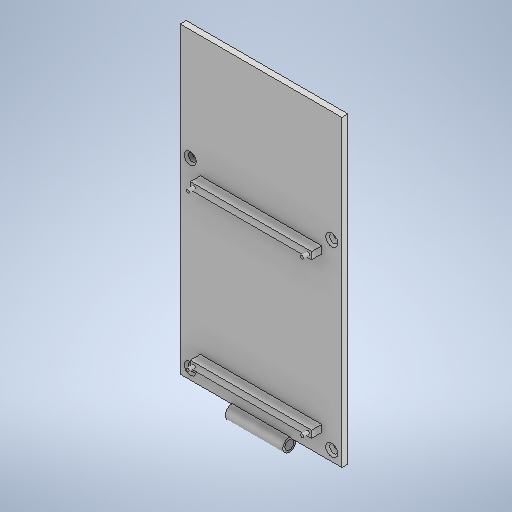
# Autodesk Inventor part: Backboard deel 1
Saved by Autodesk Inventor 2025.2 (Build 292293000, 293)
## iProperties
Created: 2024-12-12
Part Number: Backboard deel 1
Material: Generic
Document SubType Name: Modeling
Designer: jurre
Density: 1 g/cm^3
Appearance: Default
Author: jurre
Autodesk Inventor part; units mm, degrees
ref_plane "YZ Plane" through (0, 0, 0) normal (1, 0, 0) x (0, 1, 0)
ref_plane "XZ Plane" through (0, 0, 0) normal (0, 1, 0) x (-1, 0, 0)
ref_plane "XY Plane" through (0, 0, 0) normal (0, 0, 1) x (1, 0, 0)
sketch "Sketch1" plane through (0, 0, 0) normal (0, 0, 1) x (1, 0, 0)
  line L0 (-54.9903, 21.6893) -> (25.0097, 21.6893)
  line L1 (25.0097, 21.6893) -> (25.0097, -78.3107)
  line L2 (25.0097, -78.3107) -> (-54.9903, -78.3107)
  line L3 (-54.9903, -78.3107) -> (-54.9903, 21.6893)
  line L4 (-44.9903, 11.6893) -> (15.0097, 11.6893)
  line L5 (15.0097, 11.6893) -> (15.0097, -68.3107)
  line L6 (15.0097, -68.3107) -> (-44.9903, -68.3107)
  line L7 (-44.9903, -68.3107) -> (-44.9903, 11.6893)
  circle A0 centre (13.2597, 9.9393) radius 0.75
  circle A1 centre (-43.2403, 9.9393) radius 0.75
  circle A2 centre (-43.2403, -66.5607) radius 0.75
  circle A3 centre (13.2597, -66.5607) radius 0.75
  line L8 (-44.9903, 11.6893) -> (15.0097, 11.6893)
  line L9 (15.0097, 11.6893) -> (15.0097, 8.1893)
  line L10 (15.0097, 8.1893) -> (-44.9903, 8.1893)
  line L11 (-44.9903, 8.1893) -> (-44.9903, 11.6893)
  line L12 (15.0097, -68.3107) -> (-44.9903, -68.3107)
  line L13 (-44.9903, -68.3107) -> (-44.9903, -64.8107)
  line L14 (-44.9903, -64.8107) -> (15.0097, -64.8107)
  line L15 (15.0097, -64.8107) -> (15.0097, -68.3107)
  circle A4 centre (-49.9903, 16.6893) radius 2
  circle A5 centre (20.0097, 16.6893) radius 2
  circle A6 centre (20.0097, -73.3107) radius 2
  circle A7 centre (-49.9903, -73.3107) radius 2
  line L16 (-54.9903, 71.6893) -> (25.0097, 71.6893)
  line L17 (25.0097, 71.6893) -> (25.0097, -78.3107)
  line L18 (25.0097, -78.3107) -> (-54.9903, -78.3107)
  line L19 (-54.9903, -78.3107) -> (-54.9903, 71.6893)
  point P0 (0, 0)
  point P1 (-14.9903, -78.3107)
  point P2 (15.0097, -64.8107)
  point P3 (25.0097, 21.6893)
  dimension "d0" = 80
  dimension "d1" = 100
  dimension "d2" = 60
  dimension "d3" = 80
  dimension "d4" = 10
  dimension "d5" = 10
  dimension "d6" = 1.5
  dimension "d7" = 1.5
  dimension "d8" = 1.5
  dimension "d9" = 1.5
  dimension "d11" = 1.75
  dimension "d12" = 1.75
  dimension "d13" = 1.75
  dimension "d14" = 1.75
  dimension "d15" = 1.75
  dimension "d16" = 1.75
  dimension "d17" = 1.75
  dimension "d18" = 1.75
  dimension "d19" = 60
  dimension "d20" = 0
  dimension "d21" = 0
  dimension "d22" = 3.5
  dimension "d23" = 60
  dimension "d24" = 0
  dimension "d25" = 3.5
  dimension "d26" = 0
  dimension "d39" = 4
  dimension "d40" = 5
  dimension "d41" = 5
  dimension "d42" = 4
  dimension "d43" = 4
  dimension "d44" = 4
  dimension "d45" = 5
  dimension "d46" = 5
  dimension "d47" = 5
  dimension "d48" = 5
  dimension "d49" = 5
  dimension "d50" = 5
  dimension "d70" = 80
  dimension "d71" = 150
  constraints: 40 end point, 10 parallel, 8 centre point, 5 horizontal, 5 perpendicular, 1 midpoint
  measures "d0" distance of L0.start L0.end
  measures "d1" distance of L0.end L1.end
  measures "d2" distance of L4.start L4.end
  measures "d3" distance of L4.end L5.end
  measures "d4" distance from line of point (-14.99, -78.311) L6
  measures "d5" distance between parallel lines of L1 L5
  measures "d6" diameter of A0
  measures "d7" diameter of A1
  measures "d8" diameter of A2
  measures "d9" diameter of A3
  measures "d11" distance from line of L4 A1.centre
  measures "d12" distance from line of L7 A1.centre
  measures "d13" distance from line of L4 A0.centre
  measures "d14" distance from line of L5 A0.centre
  measures "d15" distance from line of L5 A3.centre
  measures "d16" distance from line of L6 A3.centre
  measures "d17" distance from line of L7 A2.centre
  measures "d18" distance from line of L6 A2.centre
  measures "d19" distance of L9.end L10.end
  measures "d20" distance between parallel lines of L5 L9
  measures "d21" distance between parallel lines of L4 L8
  measures "d22" distance of L10.end L8.start
  measures "d23" distance of L13.end L14.end
  measures "d24" distance between parallel lines of L5 L15
  measures "d25" distance of L14.end L12.start
  measures "d26" distance between parallel lines of L6 L12
  measures "d39" diameter of A4
  measures "d40" distance from line of L0 A4.centre
  measures "d41" distance from line of L3 A4.centre
  measures "d42" diameter of A5
  measures "d43" diameter of A6
  measures "d44" diameter of A7
  measures "d45" distance from line of L0 A5.centre
  measures "d46" distance from line of L1 A5.centre
  measures "d47" distance from line of L1 A6.centre
  measures "d48" distance from line of L2 A6.centre
  measures "d49" distance from line of L3 A7.centre
  measures "d50" distance from line of L2 A7.centre
  measures "d70" distance of L16.start L16.end
  measures "d71" distance of L16.end L1.end
extrude "Extrusion5" add sketch "Sketch1" against normal blind 3 contours L0 L1 L2 L3 | L4 L5 L10 L7 | L10 L5 L14 L7 | L14 L5 L6 L7 | A0 | A1 | A2 | A3 | A4 | A5 | A6 | A7
extrude "Extrusion6" cut sketch "Sketch1" against normal blind 3 contours A4 | A5 | A6 | A7
extrude "Extrusion7" add sketch "Sketch1" along normal blind 5 contours L4 L5 L10 L7 | L14 L5 L6 L7 | A0 | A1 | A2 | A3
extrude "Extrusion8" add sketch "Sketch1" along normal blind 8 contours A0 | A1 | A2 | A3
sketch "Sketch3" plane through (25.0097, -78.3107, -3) normal (1, 0, 0) x (0, 0, -1)
  circle A0 centre (-3.25, -3) radius 3.25
  line L0 (-3, 0) -> (0, 0) projected
  line L1 (-3, 0) -> (-3, 100) projected
  circle A1 centre (-3.25, -3) radius 2.25
  line L2 (0, 100) -> (0, 0) projected
  point P0 (-3, 78.3107)
  point P1 (-3, 99)
  dimension "d60" = 6.5
  dimension "d61" = 3
  dimension "d63" = 4.5
  dimension "d64" = 3.25
  constraints: 2 centre point, 1 coincident
  measures "d60" diameter of A0
  measures "d61" distance from line of L0 A0.centre
  measures "d63" diameter of A1
  measures "d64" distance from line of L2 A0.centre
extrude "Extrusion9" add sketch "Sketch3" along normal blind 28.5 separate body
move or copy body "Move Body1" bodies to move or copy 2 copy no translate (-54.25, 0, 0)
combine bodies "Combine1" operation type add bodies to combine 1 2
extrude "Extrusion10" add sketch "Sketch1" against normal blind 3 contours L19 L16 L17 L0 bodies 1
fillet "Fillet2" radius 1 4 edges at (-51.9903, 16.6893, 0) (18.0097, 16.6893, 0) (-51.9903, -73.3107, 0) (18.0097, -73.3107, 0)
body "Solid2"
